Autodesk Fusion 360 part; units mm, degrees
(part 2 of 4)
sketch "Sketch10" plane through (0, 0, 17.7) normal (0, 0, 1) x (-1, 0, 0) in component "GNSS_Enclosure_Top"
  line L0 (-53, -8.5) -> (53, -8.5)
  line L1 (-20.2661, 33.2143) -> (-20.2661, 35.8128)
  line L2 (-20.2661, 35.8128) -> (-19.6706, 35.8128)
  line L3 (-19.6706, 35.8128) -> (-19.6706, 33.2294)
  spline S0 degree 3 poles (-19.6706, 33.2294) (-19.6706, 32.473) (-19.1109, 31.8735) (-18.3752, 31.8735) knots 0 0 0 0 1 1 1 1
  spline S1 degree 3 poles (-18.3752, 31.8735) (-17.6395, 31.8735) (-17.0687, 32.4724) (-17.0687, 33.2294) knots 0 0 0 0 1 1 1 1
  line L4 (-17.0687, 33.2294) -> (-17.0687, 35.8107)
  line L5 (-17.0687, 35.8107) -> (-16.4822, 35.8107)
  line L6 (-16.4822, 35.8107) -> (-16.4822, 33.2294)
  spline S2 degree 3 poles (-16.4822, 33.2294) (-16.4822, 32.473) (-15.9046, 31.8735) (-15.1758, 31.8735) knots 0 0 0 0 1 1 1 1
  spline S3 degree 3 poles (-15.1758, 31.8735) (-14.4469, 31.8735) (-13.8755, 32.473) (-13.8755, 33.2294) knots 0 0 0 0 1 1 1 1
  line L7 (-13.8755, 33.2294) -> (-13.8755, 35.8107)
  line L8 (-13.8755, 35.8107) -> (-13.2979, 35.8107)
  line L9 (-13.2979, 35.8107) -> (-13.2979, 31.4079)
  line L10 (-13.2979, 31.4079) -> (-13.8755, 31.4079)
  line L11 (-13.8755, 31.4079) -> (-13.8755, 32.0605)
  spline S4 degree 3 poles (-13.8755, 32.0605) (-14.2016, 31.6114) (-14.7212, 31.3436) (-15.2762, 31.3385) knots 0 0 0 0 1 1 1 1
  spline S5 degree 3 poles (-15.2762, 31.3385) (-15.9326, 31.3381) (-16.5356, 31.7006) (-16.8432, 32.2805) knots 0 0 0 0 1 1 1 1
  spline S6 degree 3 poles (-16.8432, 32.2805) (-17.1409, 31.7167) (-17.7371, 31.3385) (-18.4715, 31.3385) knots 0 0 0 0 1 1 1 1
  spline S7 degree 3 poles (-18.4715, 31.3385) (-19.4953, 31.3378) (-20.2661, 32.1657) (-20.2661, 33.2143) knots 0 0 0 0 1 1 1 1
  line L12 (-25.0333, 34.1831) -> (-25.5229, 34.3592)
  spline S8 degree 3 poles (-25.5229, 34.3592) (-25.2953, 34.978) (-24.5341, 35.8478) (-23.3521, 35.8396) knots 0 0 0 0 1 1 1 1
  spline S9 degree 3 poles (-23.3521, 35.8396) (-22.3516, 35.8248) (-21.4748, 35.1666) (-21.1813, 34.2099) knots 0 0 0 0 1 1 1 1
  spline S10 degree 3 poles (-21.1813, 34.2099) (-21.121, 34.0032) (-21.0913, 33.7886) (-21.0933, 33.5732) knots 0 0 0 0 1 1 1 1
  spline S11 degree 3 poles (-21.0933, 33.5732) (-21.0779, 32.3729) (-22.0065, 31.3713) (-23.2046, 31.2961) knots 0 0 0 0 1 1 1 1
  spline S12 degree 3 poles (-23.2046, 31.2961) (-24.4027, 31.2209) (-25.4492, 32.0985) (-25.5841, 33.2913) knots 0 0 0 0 1 1 1 1
  spline S13 degree 3 poles (-25.5841, 33.2913) (-25.5912, 33.3289) (-25.5942, 33.3672) (-25.593, 33.4054) knots 0 0 0 0 1 1 1 1
  line L13 (-25.593, 33.4054) -> (-21.7679, 34.1041)
  spline S14 degree 3 poles (-21.7679, 34.1041) (-21.9694, 34.811) (-22.6142, 35.2994) (-23.3493, 35.3019) knots 0 0 0 0 1 1 1 1
  spline S15 degree 3 poles (-23.3493, 35.3019) (-24.1745, 35.3019) (-24.8318, 34.738) (-25.0333, 34.1831) knots 0 0 0 0 1 1 1 1
  spline S16 degree 3 poles (-21.6716, 33.4268) (-21.6716, 33.4797) (-21.6798, 33.5416) (-21.6798, 33.633) knots 0 0 0 0 1 1 1 1
  line L14 (-21.6798, 33.633) -> (-24.9363, 33.0431)
  spline S17 degree 3 poles (-24.9363, 33.0431) (-24.7144, 32.3251) (-24.0506, 31.8356) (-23.2992, 31.8356) knots 0 0 0 0 1 1 1 1
  spline S18 degree 3 poles (-23.2992, 31.8356) (-22.4248, 31.8593) (-21.7158, 32.5518) (-21.6716, 33.4254) knots 0 0 0 0 1 1 1 1
  line L15 (-21.6716, 33.4254) -> (-21.6716, 33.4268)
  line L16 (-30.8656, 31.4079) -> (-30.8656, 35.8128)
  line L17 (-30.8656, 35.8128) -> (-30.288, 35.8128)
  line L18 (-30.288, 35.8128) -> (-30.288, 35.099)
  spline S19 degree 3 poles (-30.288, 35.099) (-29.5994, 35.8815) (-28.4658, 36.0931) (-27.5413, 35.6116) knots 0 0 0 0 1 1 1 1
  spline S20 degree 3 poles (-27.5413, 35.6116) (-26.6169, 35.1302) (-26.1404, 34.08) (-26.3868, 33.0672) knots 0 0 0 0 1 1 1 1
  spline S21 degree 3 poles (-26.3868, 33.0672) (-26.6333, 32.0545) (-27.5391, 31.3407) (-28.5814, 31.3378) knots 0 0 0 0 1 1 1 1
  spline S22 degree 3 poles (-28.5814, 31.3378) (-29.238, 31.3347) (-29.8625, 31.6216) (-30.288, 32.1217) knots 0 0 0 0 1 1 1 1
  line L19 (-30.288, 32.1217) -> (-30.288, 31.4079)
  line L20 (-30.288, 31.4079) -> (-30.8656, 31.4079)
  spline S23 degree 3 poles (-30.2708, 33.6083) (-30.2708, 32.6456) (-29.5351, 31.8893) (-28.5896, 31.8893) knots 0 0 0 0 1 1 1 1
  spline S24 degree 3 poles (-28.5896, 31.8893) (-27.6402, 31.8893) (-26.8706, 32.6589) (-26.8706, 33.6083) knots 0 0 0 0 1 1 1 1
  spline S25 degree 3 poles (-26.8706, 33.6083) (-26.8706, 34.5577) (-27.6402, 35.3273) (-28.5896, 35.3273) knots 0 0 0 0 1 1 1 1
  spline S26 degree 3 poles (-28.5896, 35.3273) (-29.5351, 35.328) (-30.2708, 34.5709) (-30.2708, 33.6104) knots 0 0 0 0 1 1 1 1
  line L21 (-30.2708, 33.6104) -> (-30.2708, 33.6083)
  line L22 (-36.3046, 29.2592) -> (-36.3046, 35.8128)
  line L23 (-36.3046, 35.8128) -> (-35.727, 35.8128)
  line L24 (-35.727, 35.8128) -> (-35.727, 35.099)
  spline S27 degree 3 poles (-35.727, 35.099) (-35.0384, 35.8815) (-33.9048, 36.0931) (-32.9803, 35.6116) knots 0 0 0 0 1 1 1 1
  spline S28 degree 3 poles (-32.9803, 35.6116) (-32.0559, 35.1302) (-31.5794, 34.08) (-31.8258, 33.0672) knots 0 0 0 0 1 1 1 1
  spline S29 degree 3 poles (-31.8258, 33.0672) (-32.0722, 32.0545) (-32.978, 31.3407) (-34.0203, 31.3378) knots 0 0 0 0 1 1 1 1
  spline S30 degree 3 poles (-34.0203, 31.3378) (-34.6769, 31.3347) (-35.3015, 31.6216) (-35.727, 32.1217) knots 0 0 0 0 1 1 1 1
  line L25 (-35.727, 32.1217) -> (-35.727, 29.2592)
  line L26 (-35.727, 29.2592) -> (-36.3046, 29.2592)
  spline S31 degree 3 poles (-35.7098, 33.6104) (-35.7098, 32.6477) (-34.974, 31.8913) (-34.0286, 31.8913) knots 0 0 0 0 1 1 1 1
  spline S32 degree 3 poles (-34.0286, 31.8913) (-33.0831, 31.8913) (-32.3391, 32.6477) (-32.3391, 33.6104) knots 0 0 0 0 1 1 1 1
  spline S33 degree 3 poles (-32.3391, 33.6104) (-32.3391, 34.573) (-33.0831, 35.3294) (-34.0286, 35.3294) knots 0 0 0 0 1 1 1 1
  spline S34 degree 3 poles (-34.0286, 35.3294) (-34.974, 35.3294) (-35.7098, 34.5709) (-35.7098, 33.6104) knots 0 0 0 0 1 1 1 1
  spline S35 degree 3 poles (-37.2445, 33.6104) (-37.2521, 32.3647) (-38.2667, 31.3603) (-39.5124, 31.3653) knots 0 0 0 0 1 1 1 1
  spline S36 degree 3 poles (-39.5124, 31.3653) (-40.7581, 31.3704) (-41.7646, 32.383) (-41.7621, 33.6287) knots 0 0 0 0 1 1 1 1
  spline S37 degree 3 poles (-41.7621, 33.6287) (-41.7595, 34.8744) (-40.749, 35.8829) (-39.5033, 35.8829) knots 0 0 0 0 1 1 1 1
  spline S38 degree 3 poles (-39.5033, 35.8829) (-38.9019, 35.8827) (-38.3254, 35.6428) (-37.9014, 35.2163) knots 0 0 0 0 1 1 1 1
  spline S39 degree 3 poles (-37.9014, 35.2163) (-37.4775, 34.7897) (-37.241, 34.2117) (-37.2445, 33.6104) knots 0 0 0 0 1 1 1 1
  spline S40 degree 3 poles (-41.1928, 33.6104) (-41.1928, 32.6477) (-40.4577, 31.8838) (-39.5122, 31.8838) knots 0 0 0 0 1 1 1 1
  spline S41 degree 3 poles (-39.5122, 31.8838) (-38.5668, 31.8838) (-37.831, 32.6505) (-37.831, 33.6104) knots 0 0 0 0 1 1 1 1
  spline S42 degree 3 poles (-37.831, 33.6104) (-37.831, 34.5703) (-38.575, 35.3294) (-39.5122, 35.3294) knots 0 0 0 0 1 1 1 1
  spline S43 degree 3 poles (-39.5122, 35.3294) (-40.4495, 35.3294) (-41.1928, 34.5709) (-41.1928, 33.6104) knots 0 0 0 0 1 1 1 1
  line L27 (-48.7784, 31.4079) -> (-47.2293, 35.8128)
  line L28 (-47.2293, 35.8128) -> (-46.6469, 35.8128)
  line L29 (-46.6469, 35.8128) -> (-45.4092, 32.1836)
  line L30 (-45.4092, 32.1836) -> (-44.1715, 35.8128)
  line L31 (-44.1715, 35.8128) -> (-43.5939, 35.8128)
  line L32 (-43.5939, 35.8128) -> (-42.0536, 31.4079)
  line L33 (-42.0536, 31.4079) -> (-42.6312, 31.4079)
  line L34 (-42.6312, 31.4079) -> (-43.8834, 34.9938)
  line L35 (-43.8834, 34.9938) -> (-45.1437, 31.4079)
  line L36 (-45.1437, 31.4079) -> (-45.6684, 31.4079)
  line L37 (-45.6684, 31.4079) -> (-46.9295, 34.9938)
  line L38 (-46.9295, 34.9938) -> (-48.1898, 31.4079)
  line L39 (-48.1898, 31.4079) -> (-48.7784, 31.4079)
  line L40 (-1.2957, 35.8073) -> (3.6551, 35.8073)
  spline S44 degree 3 poles (3.6551, 35.8073) (3.767, 35.8073) (3.8693, 35.7438) (3.9191, 35.6436) knots 0 0 0 0 1 1 1 1
  spline S45 degree 3 poles (3.9191, 35.6436) (3.969, 35.5429) (3.9586, 35.4228) (3.8923, 35.3321) knots 0 0 0 0 1 1 1 1
  line L41 (3.8923, 35.3321) -> (-1.1369, 28.5028)
  spline S46 degree 3 poles (-1.1369, 28.5028) (-1.1924, 28.4273) (-1.2804, 28.3826) (-1.3741, 28.3825) knots 0 0 0 0 1 1 1 1
  spline S47 degree 3 poles (-1.3741, 28.3825) (-1.4668, 28.3835) (-1.5537, 28.4281) (-1.6086, 28.5028) knots 0 0 0 0 1 1 1 1
  line L42 (-1.6086, 28.5028) -> (-4.084, 31.8645)
  spline S48 degree 3 poles (-4.084, 31.8645) (-4.1812, 31.9966) (-4.1535, 32.1824) (-4.0221, 32.2805) knots 0 0 0 0 1 1 1 1
  spline S49 degree 3 poles (-4.0221, 32.2805) (-3.9594, 32.3275) (-3.8805, 32.3474) (-3.803, 32.3359) knots 0 0 0 0 1 1 1 1
  spline S50 degree 3 poles (-3.803, 32.3359) (-3.7256, 32.3244) (-3.6559, 32.2824) (-3.6095, 32.2193) knots 0 0 0 0 1 1 1 1
  line L43 (-3.6095, 32.2193) -> (-1.3741, 29.1794)
  line L44 (-1.3741, 29.1794) -> (3.0671, 35.2118)
  line L45 (3.0671, 35.2118) -> (-1.2957, 35.2118)
  spline S51 degree 3 poles (-1.2957, 35.2118) (-1.4602, 35.2118) (-1.5935, 35.3451) (-1.5935, 35.5095) knots 0 0 0 0 1 1 1 1
  spline S52 degree 3 poles (-1.5935, 35.5095) (-1.5935, 35.674) (-1.4602, 35.8073) (-1.2957, 35.8073) knots 0 0 0 0 1 1 1 1
  spline S53 degree 3 poles (-11.3527, 35.8073) (-11.2587, 35.8073) (-11.1704, 35.7626) (-11.1148, 35.6869) knots 0 0 0 0 1 1 1 1
  line L46 (-11.1148, 35.6869) -> (-6.3242, 29.1794)
  line L47 (-6.3242, 29.1794) -> (-1.5336, 35.6869)
  spline S54 degree 3 poles (-1.5336, 35.6869) (-1.4366, 35.8176) (-1.2522, 35.8453) (-1.1211, 35.7488) knots 0 0 0 0 1 1 1 1
  spline S55 degree 3 poles (-1.1211, 35.7488) (-0.9901, 35.65) (-0.9628, 35.4644) (-1.0599, 35.3321) knots 0 0 0 0 1 1 1 1
  line L48 (-1.0599, 35.3321) -> (-6.087, 28.5028)
  spline S56 degree 3 poles (-6.087, 28.5028) (-6.1424, 28.4273) (-6.2305, 28.3827) (-6.3242, 28.3827) knots 0 0 0 0 1 1 1 1
  spline S57 degree 3 poles (-6.3242, 28.3827) (-6.4179, 28.3827) (-6.506, 28.4273) (-6.5614, 28.5028) knots 0 0 0 0 1 1 1 1
  line L49 (-6.5614, 28.5028) -> (-11.5892, 35.3321)
  spline S58 degree 3 poles (-11.5892, 35.3321) (-11.6866, 35.4643) (-11.6593, 35.6502) (-11.528, 35.7488) knots 0 0 0 0 1 1 1 1
  spline S59 degree 3 poles (-11.528, 35.7488) (-11.4774, 35.7867) (-11.4159, 35.8072) (-11.3527, 35.8073) knots 0 0 0 0 1 1 1 1
  spline S60 degree 3 poles (-4.4835, 34.8584) (-4.4585, 34.8301) (-4.4229, 34.8134) (-4.3852, 34.8121) knots 0 0 0 0 1 1 1 1
  spline S61 degree 3 poles (-4.3852, 34.8121) (-4.3475, 34.8108) (-4.311, 34.825) (-4.2841, 34.8515) knots 0 0 0 0 1 1 1 1
  line L50 (-4.2841, 34.8515) -> (-4.2779, 34.8584)
  line L51 (-4.2779, 34.8584) -> (-3.5861, 35.546)
  spline S62 degree 3 poles (-3.5861, 35.546) (-3.5582, 35.5705) (-3.5413, 35.6054) (-3.5395, 35.6426) knots 0 0 0 0 1 1 1 1
  spline S63 degree 3 poles (-3.5395, 35.6426) (-3.5377, 35.6798) (-3.5511, 35.7161) (-3.5765, 35.7433) knots 0 0 0 0 1 1 1 1
  spline S64 degree 3 poles (-3.5765, 35.7433) (-3.5794, 35.7469) (-3.5826, 35.7501) (-3.5861, 35.7529) knots 0 0 0 0 1 1 1 1
  spline S65 degree 3 poles (-3.5861, 35.7529) (-3.6103, 35.7804) (-3.6445, 35.797) (-3.681, 35.7992) knots 0 0 0 0 1 1 1 1
  spline S66 degree 3 poles (-3.681, 35.7992) (-3.7175, 35.8014) (-3.7534, 35.789) (-3.7807, 35.7646) knots 0 0 0 0 1 1 1 1
  line L52 (-3.7807, 35.7646) -> (-3.7917, 35.7529)
  line L53 (-3.7917, 35.7529) -> (-4.3803, 35.1664)
  line L54 (-4.3803, 35.1664) -> (-4.9696, 35.7529)
  spline S67 degree 3 poles (-4.9696, 35.7529) (-4.9964, 35.7807) (-5.0335, 35.7959) (-5.0721, 35.7949) knots 0 0 0 0 1 1 1 1
  spline S68 degree 3 poles (-5.0721, 35.7949) (-5.1105, 35.7944) (-5.1473, 35.7794) (-5.1752, 35.7529) knots 0 0 0 0 1 1 1 1
  spline S69 degree 3 poles (-5.1752, 35.7529) (-5.2317, 35.7008) (-5.236, 35.613) (-5.1848, 35.5556) knots 0 0 0 0 1 1 1 1
  line L55 (-5.1848, 35.5556) -> (-5.1752, 35.546)
  line L56 (-5.1752, 35.546) -> (-4.4835, 34.8584)
  spline S70 degree 3 poles (-4.4835, 34.0972) (-4.4584, 34.069) (-4.4228, 34.0524) (-4.3851, 34.0512) knots 0 0 0 0 1 1 1 1
  spline S71 degree 3 poles (-4.3851, 34.0512) (-4.3474, 34.0501) (-4.3109, 34.0644) (-4.2841, 34.091) knots 0 0 0 0 1 1 1 1
  line L57 (-4.2841, 34.091) -> (-4.2779, 34.0972)
  line L58 (-4.2779, 34.0972) -> (-3.5861, 34.7889)
  spline S72 degree 3 poles (-3.5861, 34.7889) (-3.5582, 34.8135) (-3.5413, 34.8483) (-3.5395, 34.8855) knots 0 0 0 0 1 1 1 1
  spline S73 degree 3 poles (-3.5395, 34.8855) (-3.5377, 34.9227) (-3.5511, 34.9591) (-3.5765, 34.9863) knots 0 0 0 0 1 1 1 1
  spline S74 degree 3 poles (-3.5765, 34.9863) (-3.5795, 34.9896) (-3.5828, 34.9928) (-3.5861, 34.9959) knots 0 0 0 0 1 1 1 1
  spline S75 degree 3 poles (-3.5861, 34.9959) (-3.6104, 35.0232) (-3.6446, 35.0397) (-3.6812, 35.0418) knots 0 0 0 0 1 1 1 1
  spline S76 degree 3 poles (-3.6812, 35.0418) (-3.7177, 35.0439) (-3.7535, 35.0313) (-3.7807, 35.0069) knots 0 0 0 0 1 1 1 1
  spline S77 degree 2 poles (-3.7807, 35.0069) (-3.7883, 35) (-3.7917, 34.9959) knots 0 0 0 1 1 1
  line L59 (-3.7917, 34.9959) -> (-4.3803, 34.4087)
  line L60 (-4.3803, 34.4087) -> (-4.9696, 34.9959)
  spline S78 degree 3 poles (-4.9696, 34.9959) (-4.9965, 35.0233) (-5.0336, 35.0383) (-5.0721, 35.0371) knots 0 0 0 0 1 1 1 1
  spline S79 degree 3 poles (-5.0721, 35.0371) (-5.1105, 35.0374) (-5.1475, 35.0226) (-5.1752, 34.9959) knots 0 0 0 0 1 1 1 1
  spline S80 degree 3 poles (-5.1752, 34.9959) (-5.2313, 34.9436) (-5.2356, 34.8561) (-5.1848, 34.7985) knots 0 0 0 0 1 1 1 1
  line L61 (-5.1848, 34.7985) -> (-5.1752, 34.7889)
  line L62 (-5.1752, 34.7889) -> (-4.4835, 34.0972)
  spline S81 degree 3 poles (-4.4835, 33.3938) (-4.4584, 33.3656) (-4.4228, 33.349) (-4.3851, 33.3478) knots 0 0 0 0 1 1 1 1
  spline S82 degree 3 poles (-4.3851, 33.3478) (-4.3474, 33.3467) (-4.3109, 33.361) (-4.2841, 33.3876) knots 0 0 0 0 1 1 1 1
  line L63 (-4.2841, 33.3876) -> (-4.2779, 33.3938)
  line L64 (-4.2779, 33.3938) -> (-3.5861, 34.0862)
  spline S83 degree 3 poles (-3.5861, 34.0862) (-3.5295, 34.1433) (-3.5295, 34.2354) (-3.5861, 34.2925) knots 0 0 0 0 1 1 1 1
  spline S84 degree 3 poles (-3.5861, 34.2925) (-3.6134, 34.32) (-3.6505, 34.3355) (-3.6893, 34.3355) knots 0 0 0 0 1 1 1 1
  spline S85 degree 3 poles (-3.6893, 34.3355) (-3.728, 34.3355) (-3.7652, 34.32) (-3.7924, 34.2925) knots 0 0 0 0 1 1 1 1
  line L65 (-3.7924, 34.2925) -> (-4.381, 33.7059)
  line L66 (-4.381, 33.7059) -> (-4.9703, 34.2925)
  spline S86 degree 3 poles (-4.9703, 34.2925) (-4.9973, 34.3197) (-5.0344, 34.3344) (-5.0727, 34.333) knots 0 0 0 0 1 1 1 1
  spline S87 degree 3 poles (-5.0727, 34.333) (-5.111, 34.333) (-5.1479, 34.3185) (-5.1759, 34.2925) knots 0 0 0 0 1 1 1 1
  spline S88 degree 3 poles (-5.1759, 34.2925) (-5.2315, 34.24) (-5.2352, 34.1527) (-5.1841, 34.0958) knots 0 0 0 0 1 1 1 1
  line L67 (-5.1841, 34.0958) -> (-5.1745, 34.0862)
  line L68 (-5.1745, 34.0862) -> (-4.4835, 33.3938)
  spline S89 degree 3 poles (-6.428, 34.8584) (-6.4035, 34.8308) (-6.3689, 34.8143) (-6.3321, 34.8124) knots 0 0 0 0 1 1 1 1
  spline S90 degree 3 poles (-6.3321, 34.8124) (-6.2952, 34.8106) (-6.2592, 34.8237) (-6.2321, 34.8487) knots 0 0 0 0 1 1 1 1
  spline S91 degree 3 poles (-6.2321, 34.8487) (-6.2285, 34.8516) (-6.2253, 34.8548) (-6.2224, 34.8584) knots 0 0 0 0 1 1 1 1
  line L69 (-6.2224, 34.8584) -> (-5.5348, 35.546)
  spline S92 degree 3 poles (-5.5348, 35.546) (-5.5068, 35.5705) (-5.49, 35.6054) (-5.4882, 35.6426) knots 0 0 0 0 1 1 1 1
  spline S93 degree 3 poles (-5.4882, 35.6426) (-5.4864, 35.6798) (-5.4997, 35.7161) (-5.5252, 35.7433) knots 0 0 0 0 1 1 1 1
  spline S94 degree 3 poles (-5.5252, 35.7433) (-5.528, 35.7469) (-5.5313, 35.7501) (-5.5348, 35.7529) knots 0 0 0 0 1 1 1 1
  spline S95 degree 3 poles (-5.5348, 35.7529) (-5.5616, 35.7807) (-5.5988, 35.7959) (-5.6373, 35.7949) knots 0 0 0 0 1 1 1 1
  spline S96 degree 3 poles (-5.6373, 35.7949) (-5.6757, 35.7944) (-5.7125, 35.7794) (-5.7404, 35.7529) knots 0 0 0 0 1 1 1 1
  line L70 (-5.7404, 35.7529) -> (-6.3283, 35.1664)
  line L71 (-6.3283, 35.1664) -> (-6.9169, 35.7529)
  spline S97 degree 3 poles (-6.9169, 35.7529) (-6.944, 35.7808) (-6.9812, 35.7966) (-7.0201, 35.7966) knots 0 0 0 0 1 1 1 1
  spline S98 degree 3 poles (-7.0201, 35.7966) (-7.0589, 35.7966) (-7.0961, 35.7808) (-7.1232, 35.7529) knots 0 0 0 0 1 1 1 1
  spline S99 degree 3 poles (-7.1232, 35.7529) (-7.1798, 35.6958) (-7.1798, 35.6038) (-7.1232, 35.5467) knots 0 0 0 0 1 1 1 1
  line L72 (-7.1232, 35.5467) -> (-6.428, 34.8584)
  spline S100 degree 3 poles (-6.428, 34.0972) (-6.4035, 34.0696) (-6.3689, 34.0531) (-6.3321, 34.0513) knots 0 0 0 0 1 1 1 1
  spline S101 degree 3 poles (-6.3321, 34.0513) (-6.2952, 34.0495) (-6.2592, 34.0625) (-6.2321, 34.0875) knots 0 0 0 0 1 1 1 1
  line L73 (-6.2321, 34.0875) -> (-6.2224, 34.0972)
  line L74 (-6.2224, 34.0972) -> (-5.5348, 34.7889)
  spline S102 degree 3 poles (-5.5348, 34.7889) (-5.493, 34.8297) (-5.4805, 34.8919) (-5.5031, 34.9458) knots 0 0 0 0 1 1 1 1
  spline S103 degree 3 poles (-5.5031, 34.9458) (-5.5257, 34.9996) (-5.5789, 35.0342) (-5.6373, 35.033) knots 0 0 0 0 1 1 1 1
  spline S104 degree 3 poles (-5.6373, 35.033) (-5.6757, 35.0333) (-5.7127, 35.0185) (-5.7404, 34.9918) knots 0 0 0 0 1 1 1 1
  line L75 (-5.7404, 34.9918) -> (-6.3283, 34.4045)
  line L76 (-6.3283, 34.4045) -> (-6.9169, 34.9918)
  spline S105 degree 3 poles (-6.9169, 34.9918) (-6.9414, 35.0193) (-6.976, 35.0359) (-7.0129, 35.0377) knots 0 0 0 0 1 1 1 1
  spline S106 degree 3 poles (-7.0129, 35.0377) (-7.0497, 35.0395) (-7.0858, 35.0264) (-7.1129, 35.0014) knots 0 0 0 0 1 1 1 1
  spline S107 degree 3 poles (-7.1129, 35.0014) (-7.1163, 34.9983) (-7.1195, 34.9951) (-7.1225, 34.9918) knots 0 0 0 0 1 1 1 1
  spline S108 degree 3 poles (-7.1225, 34.9918) (-7.1791, 34.9347) (-7.1791, 34.8426) (-7.1225, 34.7855) knots 0 0 0 0 1 1 1 1
  line L77 (-7.1225, 34.7855) -> (-6.428, 34.0972)
  spline S109 degree 3 poles (-6.428, 33.3938) (-6.4035, 33.3662) (-6.3689, 33.3497) (-6.3321, 33.3478) knots 0 0 0 0 1 1 1 1
  spline S110 degree 3 poles (-6.3321, 33.3478) (-6.2952, 33.346) (-6.2592, 33.3591) (-6.2321, 33.3841) knots 0 0 0 0 1 1 1 1
  spline S111 degree 3 poles (-6.2321, 33.3841) (-6.2287, 33.3872) (-6.2255, 33.3904) (-6.2224, 33.3938) knots 0 0 0 0 1 1 1 1
  line L78 (-6.2224, 33.3938) -> (-5.5348, 34.0862)
  spline S112 degree 3 poles (-5.5348, 34.0862) (-5.5068, 34.1107) (-5.49, 34.1456) (-5.4882, 34.1828) knots 0 0 0 0 1 1 1 1
  spline S113 degree 3 poles (-5.4882, 34.1828) (-5.4864, 34.22) (-5.4997, 34.2563) (-5.5252, 34.2835) knots 0 0 0 0 1 1 1 1
  spline S114 degree 3 poles (-5.5252, 34.2835) (-5.5282, 34.2869) (-5.5314, 34.2901) (-5.5348, 34.2931) knots 0 0 0 0 1 1 1 1
  spline S115 degree 3 poles (-5.5348, 34.2931) (-5.5622, 34.3198) (-5.5991, 34.3344) (-5.6373, 34.3337) knots 0 0 0 0 1 1 1 1
  spline S116 degree 3 poles (-5.6373, 34.3337) (-5.6755, 34.3337) (-5.7124, 34.3192) (-5.7404, 34.2931) knots 0 0 0 0 1 1 1 1
  line L79 (-5.7404, 34.2931) -> (-6.3166, 33.7066)
  line L80 (-6.3166, 33.7066) -> (-6.9032, 34.2931)
  spline S117 degree 3 poles (-6.9032, 34.2931) (-6.9304, 34.3207) (-6.9675, 34.3362) (-7.0063, 34.3362) knots 0 0 0 0 1 1 1 1
  spline S118 degree 3 poles (-7.0063, 34.3362) (-7.045, 34.3362) (-7.0822, 34.3207) (-7.1094, 34.2931) knots 0 0 0 0 1 1 1 1
  spline S119 degree 3 poles (-7.1094, 34.2931) (-7.1653, 34.2357) (-7.1653, 34.1443) (-7.1094, 34.0869) knots 0 0 0 0 1 1 1 1
  line L81 (-7.1094, 34.0869) -> (-6.428, 33.3938)
  spline S120 degree 3 poles (-8.3712, 34.8584) (-8.3467, 34.8308) (-8.3121, 34.8143) (-8.2752, 34.8124) knots 0 0 0 0 1 1 1 1
  spline S121 degree 3 poles (-8.2752, 34.8124) (-8.2384, 34.8106) (-8.2023, 34.8237) (-8.1752, 34.8487) knots 0 0 0 0 1 1 1 1
  line L82 (-8.1752, 34.8487) -> (-8.1656, 34.8584)
  line L83 (-8.1656, 34.8584) -> (-7.478, 35.546)
  spline S122 degree 3 poles (-7.478, 35.546) (-7.45, 35.5705) (-7.4332, 35.6054) (-7.4314, 35.6426) knots 0 0 0 0 1 1 1 1
  spline S123 degree 3 poles (-7.4314, 35.6426) (-7.4296, 35.6798) (-7.4429, 35.7161) (-7.4684, 35.7433) knots 0 0 0 0 1 1 1 1
  spline S124 degree 3 poles (-7.4684, 35.7433) (-7.4712, 35.7469) (-7.4745, 35.7501) (-7.478, 35.7529) knots 0 0 0 0 1 1 1 1
  spline S125 degree 3 poles (-7.478, 35.7529) (-7.5022, 35.7804) (-7.5363, 35.797) (-7.5729, 35.7992) knots 0 0 0 0 1 1 1 1
  spline S126 degree 3 poles (-7.5729, 35.7992) (-7.6094, 35.8014) (-7.6453, 35.789) (-7.6726, 35.7646) knots 0 0 0 0 1 1 1 1
  line L84 (-7.6726, 35.7646) -> (-7.6836, 35.7529)
  line L85 (-7.6836, 35.7529) -> (-8.2722, 35.1664)
  line L86 (-8.2722, 35.1664) -> (-8.8553, 35.7591)
  spline S127 degree 3 poles (-8.8553, 35.7591) (-8.8823, 35.7863) (-8.9194, 35.801) (-8.9577, 35.7997) knots 0 0 0 0 1 1 1 1
  spline S128 degree 3 poles (-8.9577, 35.7997) (-8.9962, 35.8005) (-9.0333, 35.7859) (-9.0609, 35.7591) knots 0 0 0 0 1 1 1 1
  spline S129 degree 3 poles (-9.0609, 35.7591) (-9.1175, 35.7063) (-9.1212, 35.6178) (-9.0691, 35.5604) knots 0 0 0 0 1 1 1 1
  line L87 (-9.0691, 35.5604) -> (-9.0609, 35.5522)
  line L88 (-9.0609, 35.5522) -> (-8.3712, 34.8584)
  spline S130 degree 3 poles (-8.3712, 34.0972) (-8.3467, 34.0696) (-8.3121, 34.0531) (-8.2752, 34.0513) knots 0 0 0 0 1 1 1 1
  spline S131 degree 3 poles (-8.2752, 34.0513) (-8.2384, 34.0495) (-8.2023, 34.0625) (-8.1752, 34.0875) knots 0 0 0 0 1 1 1 1
  spline S132 degree 3 poles (-8.1752, 34.0875) (-8.1724, 34.0911) (-8.1691, 34.0943) (-8.1656, 34.0972) knots 0 0 0 0 1 1 1 1
  line L89 (-8.1656, 34.0972) -> (-7.478, 34.7889)
  spline S133 degree 3 poles (-7.478, 34.7889) (-7.45, 34.8135) (-7.4332, 34.8483) (-7.4314, 34.8855) knots 0 0 0 0 1 1 1 1
  spline S134 degree 3 poles (-7.4314, 34.8855) (-7.4296, 34.9227) (-7.4429, 34.9591) (-7.4684, 34.9863) knots 0 0 0 0 1 1 1 1
  spline S135 degree 3 poles (-7.4684, 34.9863) (-7.4714, 34.9896) (-7.4746, 34.9928) (-7.478, 34.9959) knots 0 0 0 0 1 1 1 1
  spline S136 degree 3 poles (-7.478, 34.9959) (-7.5047, 35.0228) (-7.5411, 35.038) (-7.5791, 35.038) knots 0 0 0 0 1 1 1 1
  spline S137 degree 3 poles (-7.5791, 35.038) (-7.617, 35.038) (-7.6534, 35.0228) (-7.6802, 34.9959) knots 0 0 0 0 1 1 1 1
  line L90 (-7.6802, 34.9959) -> (-7.6836, 34.9959)
  line L91 (-7.6836, 34.9959) -> (-8.2722, 34.4087)
  line L92 (-8.2722, 34.4087) -> (-8.8553, 34.9959)
  spline S138 degree 3 poles (-8.8553, 34.9959) (-8.8822, 35.0233) (-8.9193, 35.0383) (-8.9577, 35.0371) knots 0 0 0 0 1 1 1 1
  spline S139 degree 3 poles (-8.9577, 35.0371) (-8.9962, 35.0377) (-9.0334, 35.0228) (-9.0609, 34.9959) knots 0 0 0 0 1 1 1 1
  spline S140 degree 3 poles (-9.0609, 34.9959) (-9.0888, 34.9713) (-9.1057, 34.9364) (-9.1075, 34.8992) knots 0 0 0 0 1 1 1 1
  spline S141 degree 3 poles (-9.1075, 34.8992) (-9.1093, 34.8621) (-9.096, 34.8257) (-9.0705, 34.7985) knots 0 0 0 0 1 1 1 1
  line L93 (-9.0705, 34.7985) -> (-9.0609, 34.7889)
  line L94 (-9.0609, 34.7889) -> (-8.3712, 34.0972)
  spline S142 degree 3 poles (-8.3712, 33.3938) (-8.3467, 33.3662) (-8.3121, 33.3497) (-8.2752, 33.3478) knots 0 0 0 0 1 1 1 1
  spline S143 degree 3 poles (-8.2752, 33.3478) (-8.2384, 33.346) (-8.2023, 33.3591) (-8.1752, 33.3841) knots 0 0 0 0 1 1 1 1
  spline S144 degree 3 poles (-8.1752, 33.3841) (-8.1722, 33.3875) (-8.169, 33.3907) (-8.1656, 33.3938) knots 0 0 0 0 1 1 1 1
  line L95 (-8.1656, 33.3938) -> (-7.478, 34.0862)
  spline S145 degree 3 poles (-7.478, 34.0862) (-7.4214, 34.1433) (-7.4214, 34.2354) (-7.478, 34.2925) knots 0 0 0 0 1 1 1 1
  spline S146 degree 3 poles (-7.478, 34.2925) (-7.5052, 34.32) (-7.5424, 34.3355) (-7.5811, 34.3355) knots 0 0 0 0 1 1 1 1
  spline S147 degree 3 poles (-7.5811, 34.3355) (-7.6199, 34.3355) (-7.657, 34.32) (-7.6843, 34.2925) knots 0 0 0 0 1 1 1 1
  line L96 (-7.6843, 34.2925) -> (-8.2729, 33.7059)
  line L97 (-8.2729, 33.7059) -> (-8.856, 34.2925)
  spline S148 degree 3 poles (-8.856, 34.2925) (-8.883, 34.3197) (-8.9201, 34.3344) (-8.9584, 34.333) knots 0 0 0 0 1 1 1 1
  spline S149 degree 3 poles (-8.9584, 34.333) (-8.9967, 34.3332) (-9.0336, 34.3187) (-9.0616, 34.2925) knots 0 0 0 0 1 1 1 1
  spline S150 degree 3 poles (-9.0616, 34.2925) (-9.0895, 34.2679) (-9.1064, 34.233) (-9.1082, 34.1958) knots 0 0 0 0 1 1 1 1
  spline S151 degree 3 poles (-9.1082, 34.1958) (-9.11, 34.1586) (-9.0966, 34.1223) (-9.0712, 34.0951) knots 0 0 0 0 1 1 1 1
  line L98 (-9.0712, 34.0951) -> (-9.0616, 34.0855)
  line L99 (-9.0616, 34.0855) -> (-8.3712, 33.3938)
  line L100 (-12.7412, 31.3041) -> (-12.7412, 31.2348)
  spline S152 degree 3 poles (-12.7412, 31.2348) (-12.6312, 31.2348) (-12.5602, 31.2117) (-12.5283, 31.1655) knots 0 0 0 0 1 1 1 1
  spline S153 degree 3 poles (-12.5283, 31.1655) (-12.4964, 31.1193) (-12.4805, 31.0148) (-12.4805, 30.8519) knots 0 0 0 0 1 1 1 1
  line L101 (-12.4805, 30.8519) -> (-12.4805, 30.3371)
  spline S154 degree 3 poles (-12.4805, 30.3371) (-12.5883, 30.4691) (-12.7236, 30.5351) (-12.8864, 30.5351) knots 0 0 0 0 1 1 1 1
  spline S155 degree 3 poles (-12.8864, 30.5351) (-13.0427, 30.5351) (-13.1769, 30.4757) (-13.2891, 30.3569) knots 0 0 0 0 1 1 1 1
  spline S156 degree 3 poles (-13.2891, 30.3569) (-13.4013, 30.238) (-13.4574, 30.095) (-13.4574, 29.9278) knots 0 0 0 0 1 1 1 1
  spline S157 degree 3 poles (-13.4574, 29.9278) (-13.4574, 29.7606) (-13.4013, 29.6181) (-13.2891, 29.5004) knots 0 0 0 0 1 1 1 1
  spline S158 degree 3 poles (-13.2891, 29.5004) (-13.1769, 29.3827) (-13.0427, 29.3238) (-12.8864, 29.3238) knots 0 0 0 0 1 1 1 1
  spline S159 degree 3 poles (-12.8864, 29.3238) (-12.7258, 29.3238) (-12.5894, 29.3909) (-12.4772, 29.5251) knots 0 0 0 0 1 1 1 1
  spline S160 degree 3 poles (-12.4772, 29.5251) (-12.4574, 29.4151) (-12.4409, 29.348) (-12.4277, 29.3238) knots 0 0 0 0 1 1 1 1
  line L102 (-12.4277, 29.3238) -> (-11.9854, 29.4063)
  line L103 (-11.9854, 29.4063) -> (-11.9854, 29.4756)
  spline S161 degree 3 poles (-11.9854, 29.4756) (-12.0954, 29.4756) (-12.1664, 29.4982) (-12.1983, 29.5433) knots 0 0 0 0 1 1 1 1
  spline S162 degree 3 poles (-12.1983, 29.5433) (-12.2302, 29.5884) (-12.2461, 29.6935) (-12.2461, 29.8585) knots 0 0 0 0 1 1 1 1
  line L104 (-12.2461, 29.8585) -> (-12.2461, 30.8519)
  spline S163 degree 3 poles (-12.2461, 30.8519) (-12.2461, 31.017) (-12.2302, 31.122) (-12.1983, 31.1671) knots 0 0 0 0 1 1 1 1
  spline S164 degree 3 poles (-12.1983, 31.1671) (-12.1664, 31.2123) (-12.0954, 31.2348) (-11.9854, 31.2348) knots 0 0 0 0 1 1 1 1
  line L105 (-11.9854, 31.2348) -> (-11.9854, 31.3041)
  line L106 (-11.9854, 31.3041) -> (-12.7412, 31.3041)
  spline S165 degree 3 poles (-12.8171, 30.4031) (-12.7423, 30.4031) (-12.6758, 30.3794) (-12.6174, 30.3321) knots 0 0 0 0 1 1 1 1
  spline S166 degree 3 poles (-12.6174, 30.3321) (-12.5591, 30.2848) (-12.5135, 30.2204) (-12.4805, 30.139) knots 0 0 0 0 1 1 1 1
  line L107 (-12.4805, 30.139) -> (-12.4805, 29.7133)
  spline S167 degree 3 poles (-12.4805, 29.7133) (-12.5135, 29.6341) (-12.5591, 29.5713) (-12.6174, 29.5251) knots 0 0 0 0 1 1 1 1
  spline S168 degree 3 poles (-12.6174, 29.5251) (-12.6758, 29.4789) (-12.7423, 29.4558) (-12.8171, 29.4558) knots 0 0 0 0 1 1 1 1
  spline S169 degree 3 poles (-12.8171, 29.4558) (-12.9381, 29.4558) (-13.0306, 29.4998) (-13.0944, 29.5878) knots 0 0 0 0 1 1 1 1
  spline S170 degree 3 poles (-13.0944, 29.5878) (-13.1582, 29.6759) (-13.1901, 29.7892) (-13.1901, 29.9278) knots 0 0 0 0 1 1 1 1
  spline S171 degree 3 poles (-13.1901, 29.9278) (-13.1901, 30.0664) (-13.1582, 30.1808) (-13.0944, 30.2711) knots 0 0 0 0 1 1 1 1
  spline S172 degree 3 poles (-13.0944, 30.2711) (-13.0306, 30.3591) (-12.9381, 30.4031) (-12.8171, 30.4031) knots 0 0 0 0 1 1 1 1
  spline S173 degree 3 poles (-14.441, 30.5351) (-14.6236, 30.5351) (-14.7804, 30.4757) (-14.9113, 30.3569) knots 0 0 0 0 1 1 1 1
  spline S174 degree 3 poles (-14.9113, 30.3569) (-15.0422, 30.238) (-15.1077, 30.095) (-15.1077, 29.9278) knots 0 0 0 0 1 1 1 1
  spline S175 degree 3 poles (-15.1077, 29.9278) (-15.1077, 29.7606) (-15.0417, 29.6187) (-14.9097, 29.502) knots 0 0 0 0 1 1 1 1
  spline S176 degree 3 poles (-14.9097, 29.502) (-14.7798, 29.3832) (-14.6236, 29.3238) (-14.441, 29.3238) knots 0 0 0 0 1 1 1 1
  spline S177 degree 3 poles (-14.441, 29.3238) (-14.2584, 29.3238) (-14.1016, 29.3827) (-13.9707, 29.5004) knots 0 0 0 0 1 1 1 1
  spline S178 degree 3 poles (-13.9707, 29.5004) (-13.8397, 29.6181) (-13.7743, 29.7606) (-13.7743, 29.9278) knots 0 0 0 0 1 1 1 1
  spline S179 degree 3 poles (-13.7743, 29.9278) (-13.7743, 30.095) (-13.8397, 30.238) (-13.9707, 30.3569) knots 0 0 0 0 1 1 1 1
  spline S180 degree 3 poles (-13.9707, 30.3569) (-14.1016, 30.4757) (-14.2584, 30.5351) (-14.441, 30.5351) knots 0 0 0 0 1 1 1 1
  spline S181 degree 3 poles (-14.441, 30.4064) (-14.3112, 30.4064) (-14.2121, 30.3613) (-14.1439, 30.2711) knots 0 0 0 0 1 1 1 1
  spline S182 degree 3 poles (-14.1439, 30.2711) (-14.0757, 30.1808) (-14.0416, 30.0664) (-14.0416, 29.9278) knots 0 0 0 0 1 1 1 1
  spline S183 degree 3 poles (-14.0416, 29.9278) (-14.0416, 29.7892) (-14.0757, 29.6748) (-14.1439, 29.5845) knots 0 0 0 0 1 1 1 1
  spline S184 degree 3 poles (-14.1439, 29.5845) (-14.2121, 29.4943) (-14.3112, 29.4492) (-14.441, 29.4492) knots 0 0 0 0 1 1 1 1
  spline S185 degree 3 poles (-14.441, 29.4492) (-14.5708, 29.4492) (-14.6698, 29.4938) (-14.738, 29.5829) knots 0 0 0 0 1 1 1 1
  spline S186 degree 3 poles (-14.738, 29.5829) (-14.8062, 29.672) (-14.8403, 29.787) (-14.8403, 29.9278) knots 0 0 0 0 1 1 1 1
  spline S187 degree 3 poles (-14.8403, 29.9278) (-14.8403, 30.0686) (-14.8062, 30.1841) (-14.738, 30.2744) knots 0 0 0 0 1 1 1 1
  spline S188 degree 3 poles (-14.738, 30.2744) (-14.6698, 30.3624) (-14.5708, 30.4064) (-14.441, 30.4064) knots 0 0 0 0 1 1 1 1
  line L108 (-15.913, 30.5384) -> (-16.1969, 29.776)
  line L109 (-16.1969, 29.776) -> (-16.5236, 30.5384)
  line L110 (-16.5236, 30.5384) -> (-16.5896, 30.5384)
  line L111 (-16.5896, 30.5384) -> (-16.923, 29.6407)
  spline S189 degree 3 poles (-16.923, 29.6407) (-16.9494, 29.568) (-16.9802, 29.5174) (-17.0154, 29.4888) knots 0 0 0 0 1 1 1 1
  spline S190 degree 3 poles (-17.0154, 29.4888) (-17.0506, 29.4602) (-17.0979, 29.4459) (-17.1573, 29.4459) knots 0 0 0 0 1 1 1 1
  line L112 (-17.1573, 29.4459) -> (-17.1573, 29.3799)
  line L113 (-17.1573, 29.3799) -> (-16.6952, 29.3799)
  line L114 (-16.6952, 29.3799) -> (-16.6952, 29.4459)
  spline S191 degree 3 poles (-16.6952, 29.4459) (-16.8053, 29.4459) (-16.8372, 29.5108) (-16.7909, 29.6407) knots 0 0 0 0 1 1 1 1
  line L115 (-16.7909, 29.6407) -> (-16.6127, 30.1555)
  line L116 (-16.6127, 30.1555) -> (-16.2761, 29.3799)
  line L117 (-16.2761, 29.3799) -> (-16.2035, 29.3799)
  line L118 (-16.2035, 29.3799) -> (-15.9361, 30.1555)
  line L119 (-15.9361, 30.1555) -> (-15.7117, 29.6407)
  spline S192 degree 3 poles (-15.7117, 29.6407) (-15.6545, 29.5108) (-15.6941, 29.4459) (-15.8305, 29.4459) knots 0 0 0 0 1 1 1 1
  line L120 (-15.8305, 29.4459) -> (-15.8305, 29.3799)
  line L121 (-15.8305, 29.3799) -> (-15.2331, 29.3799)
  line L122 (-15.2331, 29.3799) -> (-15.2331, 29.4459)
  spline S193 degree 3 poles (-15.2331, 29.4459) (-15.2837, 29.4459) (-15.3261, 29.4602) (-15.3602, 29.4888) knots 0 0 0 0 1 1 1 1
  spline S194 degree 3 poles (-15.3602, 29.4888) (-15.3943, 29.5174) (-15.4267, 29.568) (-15.4575, 29.6407) knots 0 0 0 0 1 1 1 1
  line L123 (-15.4575, 29.6407) -> (-15.847, 30.5384)
  line L124 (-15.847, 30.5384) -> (-15.913, 30.5384)
  spline S195 degree 3 poles (-17.8768, 30.5351) (-17.9692, 30.5351) (-18.0616, 30.5147) (-18.1541, 30.474) knots 0 0 0 0 1 1 1 1
  spline S196 degree 3 poles (-18.1541, 30.474) (-18.2465, 30.4333) (-18.3224, 30.3811) (-18.3818, 30.3173) knots 0 0 0 0 1 1 1 1
  line L125 (-18.3818, 30.3173) -> (-18.3224, 30.2447)
  spline S197 degree 3 poles (-18.3224, 30.2447) (-18.2762, 30.2887) (-18.2179, 30.325) (-18.1475, 30.3536) knots 0 0 0 0 1 1 1 1
  spline S198 degree 3 poles (-18.1475, 30.3536) (-18.0771, 30.3822) (-18.0143, 30.3965) (-17.9593, 30.3965) knots 0 0 0 0 1 1 1 1
  spline S199 degree 3 poles (-17.9593, 30.3965) (-17.7965, 30.3965) (-17.6793, 30.3453) (-17.6078, 30.243) knots 0 0 0 0 1 1 1 1
  spline S200 degree 3 poles (-17.6078, 30.243) (-17.5363, 30.1407) (-17.5105, 30.0081) (-17.5303, 29.8453) knots 0 0 0 0 1 1 1 1
  line L126 (-17.5303, 29.8453) -> (-18.3257, 29.8453)
  spline S201 degree 3 poles (-18.3257, 29.8453) (-18.3653, 29.7067) (-18.3378, 29.5851) (-18.2432, 29.4806) knots 0 0 0 0 1 1 1 1
  spline S202 degree 3 poles (-18.2432, 29.4806) (-18.1486, 29.3761) (-18.0264, 29.3238) (-17.8768, 29.3238) knots 0 0 0 0 1 1 1 1
  spline S203 degree 3 poles (-17.8768, 29.3238) (-17.7184, 29.3238) (-17.577, 29.3821) (-17.4527, 29.4987) knots 0 0 0 0 1 1 1 1
  spline S204 degree 3 poles (-17.4527, 29.4987) (-17.3284, 29.6154) (-17.2662, 29.7584) (-17.2662, 29.9278) knots 0 0 0 0 1 1 1 1
  spline S205 degree 3 poles (-17.2662, 29.9278) (-17.2662, 30.0972) (-17.3234, 30.2408) (-17.4379, 30.3585) knots 0 0 0 0 1 1 1 1
  spline S206 degree 3 poles (-17.4379, 30.3585) (-17.5523, 30.4762) (-17.6986, 30.5351) (-17.8768, 30.5351) knots 0 0 0 0 1 1 1 1
  line L127 (-18.098, 29.7232) -> (-17.5501, 29.7232)
  spline S207 degree 3 poles (-17.5501, 29.7232) (-17.5743, 29.6418) (-17.6144, 29.5768) (-17.6705, 29.5284) knots 0 0 0 0 1 1 1 1
  spline S208 degree 3 poles (-17.6705, 29.5284) (-17.7266, 29.48) (-17.7899, 29.4558) (-17.8603, 29.4558) knots 0 0 0 0 1 1 1 1
  spline S209 degree 3 poles (-17.8603, 29.4558) (-17.9593, 29.4558) (-18.0292, 29.485) (-18.0699, 29.5433) knots 0 0 0 0 1 1 1 1
  spline S210 degree 3 poles (-18.0699, 29.5433) (-18.1106, 29.6016) (-18.12, 29.6616) (-18.098, 29.7232) knots 0 0 0 0 1 1 1 1
  line L128 (-19.3819, 30.479) -> (-19.3819, 30.4097)
  spline S211 degree 3 poles (-19.3819, 30.4097) (-19.2718, 30.4097) (-19.2009, 30.3866) (-19.169, 30.3404) knots 0 0 0 0 1 1 1 1
  spline S212 degree 3 poles (-19.169, 30.3404) (-19.1371, 30.2942) (-19.1211, 30.1885) (-19.1211, 30.0235) knots 0 0 0 0 1 1 1 1
  line L129 (-19.1211, 30.0235) -> (-19.1211, 29.842)
  spline S213 degree 3 poles (-19.1211, 29.842) (-19.1211, 29.7254) (-19.1508, 29.6319) (-19.2102, 29.5614) knots 0 0 0 0 1 1 1 1
  spline S214 degree 3 poles (-19.2102, 29.5614) (-19.2696, 29.491) (-19.3246, 29.4558) (-19.3753, 29.4558) knots 0 0 0 0 1 1 1 1
  spline S215 degree 3 poles (-19.3753, 29.4558) (-19.4457, 29.4558) (-19.4809, 29.4921) (-19.4809, 29.5647) knots 0 0 0 0 1 1 1 1
  spline S216 degree 3 poles (-19.4809, 29.5647) (-19.4809, 29.5955) (-19.4924, 29.6231) (-19.5155, 29.6473) knots 0 0 0 0 1 1 1 1
  spline S217 degree 3 poles (-19.5155, 29.6473) (-19.5386, 29.6715) (-19.5656, 29.6836) (-19.5964, 29.6836) knots 0 0 0 0 1 1 1 1
  spline S218 degree 3 poles (-19.5964, 29.6836) (-19.6844, 29.6836) (-19.7284, 29.6319) (-19.7284, 29.5284) knots 0 0 0 0 1 1 1 1
  spline S219 degree 3 poles (-19.7284, 29.5284) (-19.7284, 29.48) (-19.7059, 29.4338) (-19.6607, 29.3898) knots 0 0 0 0 1 1 1 1
  spline S220 degree 3 poles (-19.6607, 29.3898) (-19.6156, 29.3458) (-19.5513, 29.3238) (-19.4677, 29.3238) knots 0 0 0 0 1 1 1 1
  spline S221 degree 3 poles (-19.4677, 29.3238) (-19.4017, 29.3238) (-19.3356, 29.3469) (-19.2696, 29.3931) knots 0 0 0 0 1 1 1 1
  spline S222 degree 3 poles (-19.2696, 29.3931) (-19.2036, 29.4393) (-19.1541, 29.4954) (-19.1211, 29.5614) knots 0 0 0 0 1 1 1 1
  spline S223 degree 3 poles (-19.1211, 29.5614) (-19.1035, 29.4448) (-19.0848, 29.3656) (-19.065, 29.3238) knots 0 0 0 0 1 1 1 1
  line L130 (-19.065, 29.3238) -> (-18.626, 29.4063)
  line L131 (-18.626, 29.4063) -> (-18.626, 29.4756)
  spline S224 degree 3 poles (-18.626, 29.4756) (-18.7361, 29.4756) (-18.807, 29.4987) (-18.8389, 29.5449) knots 0 0 0 0 1 1 1 1
  spline S225 degree 3 poles (-18.8389, 29.5449) (-18.8708, 29.5911) (-18.8868, 29.6957) (-18.8868, 29.8585) knots 0 0 0 0 1 1 1 1
  line L132 (-18.8868, 29.8585) -> (-18.8868, 30.0235)
  spline S226 degree 3 poles (-18.8868, 30.0235) (-18.8868, 30.1885) (-18.8708, 30.2942) (-18.8389, 30.3404) knots 0 0 0 0 1 1 1 1
  spline S227 degree 3 poles (-18.8389, 30.3404) (-18.807, 30.3866) (-18.7361, 30.4097) (-18.626, 30.4097) knots 0 0 0 0 1 1 1 1
  line L133 (-18.626, 30.4097) -> (-18.626, 30.479)
  line L134 (-18.626, 30.479) -> (-19.3819, 30.479)
  spline S228 degree 3 poles (-20.5667, 30.5351) (-20.6592, 30.5351) (-20.7516, 30.5147) (-20.844, 30.474) knots 0 0 0 0 1 1 1 1
  spline S229 degree 3 poles (-20.844, 30.474) (-20.9364, 30.4333) (-21.0123, 30.3811) (-21.0717, 30.3173) knots 0 0 0 0 1 1 1 1
  line L135 (-21.0717, 30.3173) -> (-21.0123, 30.2447)
  spline S230 degree 3 poles (-21.0123, 30.2447) (-20.9661, 30.2887) (-20.9078, 30.325) (-20.8374, 30.3536) knots 0 0 0 0 1 1 1 1
  spline S231 degree 3 poles (-20.8374, 30.3536) (-20.767, 30.3822) (-20.7043, 30.3965) (-20.6493, 30.3965) knots 0 0 0 0 1 1 1 1
  spline S232 degree 3 poles (-20.6493, 30.3965) (-20.4864, 30.3965) (-20.3693, 30.3453) (-20.2977, 30.243) knots 0 0 0 0 1 1 1 1
  spline S233 degree 3 poles (-20.2977, 30.243) (-20.2262, 30.1407) (-20.2004, 30.0081) (-20.2202, 29.8453) knots 0 0 0 0 1 1 1 1
  line L136 (-20.2202, 29.8453) -> (-21.0156, 29.8453)
  spline S234 degree 3 poles (-21.0156, 29.8453) (-21.0552, 29.7067) (-21.0277, 29.5851) (-20.9331, 29.4806) knots 0 0 0 0 1 1 1 1
  spline S235 degree 3 poles (-20.9331, 29.4806) (-20.8385, 29.3761) (-20.7164, 29.3238) (-20.5667, 29.3238) knots 0 0 0 0 1 1 1 1
  spline S236 degree 3 poles (-20.5667, 29.3238) (-20.4083, 29.3238) (-20.2669, 29.3821) (-20.1426, 29.4987) knots 0 0 0 0 1 1 1 1
  spline S237 degree 3 poles (-20.1426, 29.4987) (-20.0183, 29.6154) (-19.9561, 29.7584) (-19.9561, 29.9278) knots 0 0 0 0 1 1 1 1
  spline S238 degree 3 poles (-19.9561, 29.9278) (-19.9561, 30.0972) (-20.0134, 30.2408) (-20.1278, 30.3585) knots 0 0 0 0 1 1 1 1